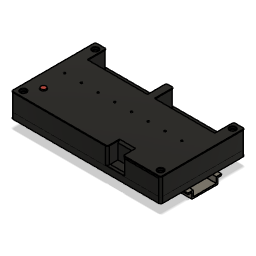
RelayBoardMount (Autodesk Fusion 360 design; units mm, degrees)
Autodesk Fusion 360 part; units mm, degrees
sketch "Skizze1" plane through (0, 0, 0) normal (1, 0, 0) x (0, 0, -1) in component "Rail"
  line L0 (-17.5, 0) -> (17.5, 0)
  line L1 (-13.5, -7.5) -> (13.5, -7.5)
  line L2 (0, -7.5) -> (0, 0) construction
  line L3 (-17.5, 0) -> (-17.5, -1.5)
  line L4 (17.5, 0) -> (17.5, -1.5)
  line L5 (13.5, -7.5) -> (13.5, -1.5)
  line L6 (13.5, -1.5) -> (17.5, -1.5)
  line L7 (-17.5, -1.5) -> (-13.5, -1.5)
  line L8 (-13.5, -1.5) -> (-13.5, -7.5)
  line L9 (-12, 0) -> (-12, -6)
  line L10 (-12, -6) -> (12, -6)
  line L11 (12, -6) -> (12, 0)
  dimension "d1" = 35
  dimension "d2" = 27
  dimension "d3" = 1.5
  dimension "d5" = 7.5
  dimension "d6" = 1.5
  dimension "d7" = 1.5
  dimension "d8" = 1.5
  constraint horizontal L0
  constraint midpoint L2.end L0
  constraint horizontal L1
  constraint midpoint L1 L2.start
  constraint coincident L2.end origin
  constraint vertical L2
  constraint perpendicular L0 L3
  constraint perpendicular L0 L4
  constraint perpendicular L1 L5
  constraint perpendicular L4 L6
  constraint perpendicular L5 L7
  constraint perpendicular L7 L8
  constraint equal L3 L4
  constraint coincident L0 L9.start
  constraint perpendicular L0 L9
  constraint perpendicular L5 L10
  constraint coincident L0 L11.end
  constraint perpendicular L0 L11
  measures "d1" distance of L0.start L0.end
  measures "d2" distance of L1.start L1.end
  measures "d3" distance of L0.end L4.end
  measures "d5" distance of L0 L1
  measures "d6" distance of L1 L10
  measures "d7" distance of L8 L9
  measures "d8" distance of L5 L11
extrude "Extrusion1" add sketch "Skizze1" along normal mid plane 160 contours L0 L1 L3 L4 L5 L6 L7 L8 L9 L10 L11 makes body 1 in component "Rail"
sketch "Skizze1 (2)" plane through (0, 0, 0) normal (0, 1, 0) x (1, 0, 0) in component "DinRailMount"
  line L0 (-80, 17.5) -> (80, 17.5)
  line L1 (-80, 12) -> (80, 12)
  line L2 (-80, -12) -> (80, -12)
  line L3 (80, -17.5) -> (-80, -17.5)
  line L4 (0, 17.5) -> (0, -17.5) construction
  line L5 (-5, 17.5) -> (5, 17.5)
  line L6 (5, 17.5) -> (5, 20.5)
  line L7 (5, 20.5) -> (-5, 20.5)
  line L8 (-5, 20.5) -> (-5, 17.5)
  arc A0 (0, 17.5) -> (0, 11.5) centre (0, 14.5) ccw
  arc A1 (0, 5.5) -> (0, 11.5) centre (0, 8.5) ccw
  arc A2 (0, 5.5) -> (0, -0.5) centre (0, 2.5) ccw
  arc A3 (0, -6.5) -> (0, -0.5) centre (0, -3.5) ccw
  arc A4 (0, -5.8) -> (0, -1.2) centre (0, -3.5) ccw
  arc A5 (0, 6.2) -> (0, -1.2) centre (0, 2.5) ccw
  arc A6 (0, 6.2) -> (0, 10.8) centre (0, 8.5) ccw
  arc A7 (0, 18.2) -> (0, 10.8) centre (0, 14.5) ccw
  arc A8 (0, 16.8) -> (0, 12.2) centre (0, 14.5) ccw
  arc A9 (0, 4.8) -> (0, 12.2) centre (0, 8.5) ccw
  arc A10 (0, 4.8) -> (0, 0.2) centre (0, 2.5) ccw
  arc A11 (0, -7.2) -> (0, 0.2) centre (0, -3.5) ccw
  arc A12 (0, 16.8) -> (5, 17.5) centre (0, 35.0071) ccw
  line L9 (-8.5, 22.5) -> (8.5, 22.5) construction
  line L10 (8.5, 22.5) -> (8.5, -20.5)
  line L11 (8.5, -20.5) -> (-8.5, -20.5)
  line L12 (-8.5, -20.5) -> (-8.5, 22.5)
  line L13 (0, -17.5) -> (0, -20.5) construction
  line L14 (-5.5, 22.5) -> (5.5, 22.5)
  line L15 (5.5, 22.5) -> (5.5, -6.5)
  line L16 (5.5, -6.5) -> (-5.5, -6.5)
  line L17 (-5.5, -6.5) -> (-5.5, 22.5)
  arc A13 (0, -5.8) -> (-5.5, -6.5) centre (0, -27.7571) ccw
  line L18 (8.5, 22.5) -> (8.5, 30.5)
  line L19 (8.5, 30.5) -> (-8.5, 30.5)
  line L20 (-8.5, 30.5) -> (-8.5, 22.5)
  line L21 (0, 30.5) -> (0, 22.5) construction
  circle A14 centre (0, 26.5) radius 1.75
  circle A15 centre (0, -9.5) radius 1.75
  dimension "d89" = 10
  dimension "d91" = 3
  dimension "d94" = 3
  dimension "d95" = 6
  dimension "d98" = 0
  dimension "d99" = -12
  dimension "d100" = 0.7
  dimension "d101" = -0.7
  dimension "d102" = 5
  dimension "d103" = 3
  dimension "d105" = 2
  dimension "d106" = 3.5
  dimension "d107" = 4
  dimension "d108" = 3
  dimension "d111" = 0.5
  dimension "d149" = 3
  constraint midpoint L0 L4.start
  constraint midpoint L3 L4.end
  constraint horizontal L5
  constraint vertical L6
  constraint horizontal L7
  constraint vertical L8
  constraint coincident L0 L5.start
  constraint midpoint L4.start L5
  constraint coincident L4 A0.end
  constraint coincident L4 A0.centre
  constraint coincident L4 A1.start
  constraint coincident L4 A1.centre
  constraint tangent A8 A12
  constraint horizontal L9
  constraint vertical L10
  constraint horizontal L11
  constraint vertical L12
  constraint midpoint L11 L13.end
  constraint collinear L4 L13
  constraint horizontal L14
  constraint vertical L15
  constraint horizontal L16
  constraint vertical L17
  constraint midpoint A3.start L16
  constraint tangent A4 A13
  constraint vertical L18
  constraint horizontal L19
  constraint vertical L20
  constraint coincident L9.end L10.start
  constraint midpoint L19 L21.start
  constraint midpoint L21 A14.centre
  constraint midpoint L14 L21.end
  constraint coincident L4 A15.centre
  constraint equal A14 A15
  measures "d89" distance of L5.start L5.end
  measures "d91" distance of L5.end L6.end
  measures "d94" distance of L5 A0.centre
  measures "d95" distance of A0.centre A1.centre
  measures "d102" distance of L0 L9
  measures "d103" distance of L3 L11
  measures "d105" distance of L7 L14
  measures "d106" diameter of A14
  measures "d107" distance of L19 A14.centre
  measures "d108" distance of L16 A15.centre
  measures "d111" distance of L8 L17
  measures "d149" distance of L12 L17
extrude "Extrusion1'" add sketch "Skizze1 (2)" along normal blind 3 separate body contours L0 L5 L6 L7 L8 | L0 L1 L5 A0 A7 | L0 L1 L5 A0 A8 A9 A12 | L1 A0 A1 A2 A3 A4 A5 A6 A7 L16 A13 | L1 A0 A1 A2 A3 A9 A10 A11 L16 | L0 L10 L12 L14 L15 L17 L18 L19 L20 | L0 L1 L10 L15 | L1 L2 L10 L12 L15 L16 L17 | L0 L1 L12 L17 | L2 L3 L10 L12 | L3 L10 L11 L12 makes body 2 in component "DinRailMount"
sketch "Skizze2" plane through (0, 3, 0) normal (0, 1, 0) x (-1, 0, 0) in component "DinRailMount"
  circle A0 centre (0, -26.5) radius 1.75
  circle A1 centre (0, 9.5) radius 1.75
  line L0 (5.5, 6.5) -> (5.5, -22.5)
  line L1 (5.5, -22.5) -> (-5.5, -22.5)
  line L2 (-5.5, -22.5) -> (-5.5, 6.5)
  line L3 (-5.5, 6.5) -> (-2.1656, 6.5)
  line L4 (-8.5, 20.5) -> (-8.5, -30.5)
  line L5 (-8.5, -30.5) -> (8.5, -30.5)
  line L6 (8.5, -30.5) -> (8.5, 20.5)
  line L7 (8.5, 20.5) -> (-8.5, 20.5)
  line L8 (5, -17.5) -> (6, -17.5)
  line L9 (6, -17.5) -> (6, -22)
  line L10 (6, -22) -> (5.5, -22)
  line L11 (5, -20.5) -> (6, -20.5)
  line L12 (5, -17) -> (6.5, -17)
  line L13 (6.5, -17) -> (6.5, -22.5)
  line L14 (6.5, -22.5) -> (5.5, -22.5)
  line L15 (-5, -17.5) -> (-6, -17.5)
  line L16 (-6, -17.5) -> (-6, -22)
  line L17 (-6, -22) -> (-5.5, -22)
  line L18 (-5, -20.5) -> (-6, -20.5)
  line L19 (-5, -17) -> (-6.5, -17)
  line L20 (-6.5, -17) -> (-6.5, -22.5)
  line L21 (-6.5, -22.5) -> (-5.5, -22.5)
  line L22 (5, -20.5) -> (5, -17.5)
  line L23 (5, -17.5) -> (2.1656, -17.5)
  line L24 (-5, -17.5) -> (-5, -20.5)
  line L25 (-5, -20.5) -> (5, -20.5)
  line L26 (-5, -17.5) -> (-5, -20.5)
  line L27 (-5, -20.5) -> (5, -20.5)
  line L28 (5, -20.5) -> (5, -17.5)
  line L29 (5, -17.5) -> (2.1656, -17.5)
  line L30 (-8.5, 20.5) -> (-8.5, -30.5)
  line L31 (-8.5, -30.5) -> (8.5, -30.5)
  line L32 (8.5, -30.5) -> (8.5, 20.5)
  line L33 (8.5, 20.5) -> (-8.5, 20.5)
  circle A2 centre (0, 9.5) radius 1.75
  circle A3 centre (0, -26.5) radius 1.75
  line L34 (5.5, 6.5) -> (5.5, -22.5)
  line L35 (5.5, -22.5) -> (-5.5, -22.5)
  line L36 (-5.5, -22.5) -> (-5.5, 6.5)
  line L37 (-5.5, 6.5) -> (-2.1656, 6.5)
  arc A4 (0, -4.8) -> (0, -12.2) centre (0, -8.5) ccw
  arc A5 (0, -16.8) -> (0, -12.2) centre (0, -14.5) ccw
  arc A6 (0, -16.8) -> (-5, -17.5) centre (0, -35.0071) ccw
  arc A7 (2.1656, -17.5) -> (0, -10.8) centre (0, -14.5) ccw
  arc A8 (0, -6.2) -> (0, -10.8) centre (0, -8.5) ccw
  arc A9 (0, -6.2) -> (0, 1.2) centre (0, -2.5) ccw
  arc A10 (0, 5.8) -> (0, 1.2) centre (0, 3.5) ccw
  arc A11 (0, 5.8) -> (5.5, 6.5) centre (0, 27.7571) ccw
  arc A12 (-2.1656, 6.5) -> (0, -0.2) centre (0, 3.5) ccw
  arc A13 (0, -4.8) -> (0, -0.2) centre (0, -2.5) ccw
  arc A14 (0, -4.8) -> (0, -12.2) centre (0, -8.5) ccw
  arc A15 (0, -16.8) -> (0, -12.2) centre (0, -14.5) ccw
  arc A16 (0, -16.8) -> (-5, -17.5) centre (0, -35.0071) ccw
  arc A17 (2.1656, -17.5) -> (0, -10.8) centre (0, -14.5) ccw
  arc A18 (0, -6.2) -> (0, -10.8) centre (0, -8.5) ccw
  arc A19 (0, -6.2) -> (0, 1.2) centre (0, -2.5) ccw
  arc A20 (0, 5.8) -> (0, 1.2) centre (0, 3.5) ccw
  arc A21 (0, 5.8) -> (5.5, 6.5) centre (0, 27.7571) ccw
  arc A22 (-2.1656, 6.5) -> (0, -0.2) centre (0, 3.5) ccw
  arc A23 (0, -4.8) -> (0, -0.2) centre (0, -2.5) ccw
  dimension "d119" = 0.5
  dimension "d120" = -0.5
  dimension "d121" = 0.5
  dimension "d148" = 0.5
  constraint perpendicular L1 L9
  constraint perpendicular L0 L10
  constraint coincident L9 L11.end
  constraint perpendicular L9 L11
  constraint coincident L0 L10.end
  constraint coincident L1 L0.end
  constraint perpendicular L2 L15
  constraint perpendicular L15 L16
  constraint coincident L2 L17.end
  constraint perpendicular L2 L17
  constraint coincident L16 L18.end
  constraint perpendicular L16 L18
  constraint equal L8 L15
  constraint equal L9 L16
  measures "d119" distance of L0 L9
  measures "d121" distance of L1 L10
extrude "Extrusion2" cut sketch "Skizze2" against normal blind 1.4 from surface at -0.5 contours L0 L8 L9 L10 L12 L13 L14 L34 | L0 L9 L10 L11 L34 | L0 L8 L9 L11 L34 | L2 L15 L16 L17 L19 L20 L21 L36 | L2 L16 L17 L18 L36 | L2 L15 L16 L18 L36 bodies 2 in component "DinRailMount"
extrude "Extrusion3" add sketch "Skizze2" along normal blind 1 from surface at -1.7 contours L0 L8 L11 L22 L28 L34 | L0 L8 L9 L11 L34 | L2 L15 L18 L24 L26 L36 | L2 L15 L16 L18 L36 bodies 2 in component "DinRailMount"
sketch "Skizze3" plane through (5, 0, 0) normal (1, 0, 0) x (0, 0, -1) in component "DinRailMount"
  line L0 (20.5, 1.3) -> (17.5, 1.3)
  line L1 (17.5, 0) -> (20.5, 0)
  line L2 (20.5, 0) -> (20.5, 1.3)
  line L3 (-17.5, 0) -> (-17.5, -1.5)
  line L4 (-17.5, -1.5) -> (-13.5, -1.5)
  line L5 (-13.5, -1.5) -> (-13.5, -7.5)
  line L6 (-13.5, -7.5) -> (13.5, -7.5)
  line L7 (13.5, -7.5) -> (13.5, -1.5)
  line L8 (13.5, -1.5) -> (17.5, -1.5)
  line L9 (17.5, -1.5) -> (17.5, 0)
  line L10 (17.5, 0) -> (12, 0)
  line L11 (12, 0) -> (12, -6)
  line L12 (12, -6) -> (-12, -6)
  line L13 (-12, -6) -> (-12, 0)
  line L14 (-12, 0) -> (-17.5, 0)
  line L15 (20.5, 0) -> (20.5, -2)
  line L16 (16, -2) -> (16, -1.5)
  line L17 (16, -2) -> (17, -3)
  line L18 (17, -3) -> (19.5, -3)
  line L19 (19.5, -3) -> (20.5, -2)
  line L20 (20.5, -2) -> (16, -2) construction
  line L21 (17.5, 1.3) -> (17.5, 0)
  dimension "d127" = 1.5
  dimension "d129" = 0.5
  dimension "d130" = 1.5
  dimension "d151" = 45
  dimension "d152" = 45
  constraint coincident L1.end L2.start
  constraint perpendicular L1 L15
  constraint coincident L8 L16.end
  constraint perpendicular L8 L16
  constraint horizontal L18
  constraint perpendicular L16 L20
  measures "d127" distance of L9 L16
  measures "d129" distance of L16.start L16.end
  measures "d130" distance of L8 L18
  measures "d151" angle of L17 L20
  measures "d152" angle of L19 L20
extrude "Extrusion4" add sketch "Skizze3" against normal up to surface (10 mm away) contours L1 L8 L9 L15 L16 L17 L18 L19 bodies 2 in component "DinRailMount"
sketch "Skizze4" plane through (8.5, 0, 0) normal (1, 0, 0) x (0, 0, -1) in component "DinRailMount"
  line L0 (-20.5, 0) -> (30.5, 0)
  line L1 (30.5, 0) -> (30.5, 3)
  line L2 (30.5, 3) -> (-20.5, 3)
  line L3 (-20.5, 3) -> (-20.5, 0)
  line L4 (-17.5, 0) -> (-17.5, -1.5)
  line L5 (-17.5, -1.5) -> (-13.5, -1.5)
  line L6 (-13.5, -1.5) -> (-13.5, -7.5)
  line L7 (-13.5, -7.5) -> (13.5, -7.5)
  line L8 (13.5, -7.5) -> (13.5, -1.5)
  line L9 (13.5, -1.5) -> (17.5, -1.5)
  line L10 (17.5, -1.5) -> (17.5, 0)
  line L11 (17.5, 0) -> (12, 0)
  line L12 (12, 0) -> (12, -6)
  line L13 (12, -6) -> (-12, -6)
  line L14 (-12, -6) -> (-12, 0)
  line L15 (-12, 0) -> (-17.5, 0)
  line L16 (-20.5, 0) -> (-20.5, -2)
  line L17 (-19.5, -3) -> (-20.5, -2)
  line L18 (-17, -3) -> (-19.5, -3)
  line L19 (-16, -2) -> (-17, -3)
  line L20 (-16, -2) -> (-16, -1.5)
  line L21 (-16, -2) -> (-20.5, -2) construction
  dimension "d141" = 0.5
  dimension "d143" = 1.5
  dimension "d144" = 1.5
  dimension "d153" = 45
  dimension "d154" = 45
  constraint coincident L0 L3.end
  constraint coincident L0.start L3.end
  constraint coincident L5 L20.end
  constraint perpendicular L5 L20
  constraint perpendicular L0 L16
  constraint perpendicular L20 L21
  measures "d141" distance of L19.start L20.end
  measures "d143" distance of L5 L18
  measures "d144" distance of L4 L20
  measures "d153" angle of L17 L21
  measures "d154" angle of L19 L21
extrude "Extrusion5" add sketch "Skizze4" against normal up to surface (17 mm away) contours L0 L4 L5 L16 L17 L18 L19 L20 bodies 2 in component "DinRailMount"
chamfer "Fase1" distance 1 angle 45 2 edges at (-1.6316, 0, -27.1328) (-1.6316, 0, 8.8672) on bodies 2 in component "DinRailMount"
ref_plane "Arbeitsebene1" through (0, 2, -5) normal (0, 1, 0) x (1, 0, 0) in component "DinRailMount"
sketch "Skizze2 (2)" plane through (0, 2, 0) normal (0, 1, 0) x (1, 0, 0) in component "RelayBottom"
  line L0 (-74, 40) -> (74, 40)
  line L1 (74, 40) -> (74, -40)
  line L2 (74, -40) -> (-74, -40)
  line L3 (-74, -40) -> (-74, 40)
  line L4 (-74, 40) -> (74, -40) construction
  line L5 (74, 40) -> (-74, -40) construction
  line L6 (-77, 43) -> (77, 43)
  line L7 (77, 43) -> (77, -43)
  line L8 (77, -43) -> (-77, -43)
  line L9 (-77, -43) -> (-77, 43)
  circle A0 centre (-71.5, 37.5) radius 2
  line L10 (71.5, -37.5) -> (-71.5, -37.5) construction
  line L11 (-71.5, -37.5) -> (-71.5, 37.5) construction
  line L12 (-71.5, 37.5) -> (71.5, 37.5) construction
  line L13 (71.5, 37.5) -> (71.5, -37.5) construction
  line L14 (71.5, -37.5) -> (-71.5, 37.5) construction
  line L15 (-71.5, -37.5) -> (71.5, 37.5) construction
  circle A1 centre (71.5, 37.5) radius 2
  circle A2 centre (71.5, -37.5) radius 2
  circle A3 centre (-71.5, -37.5) radius 2
  line L16 (-68.5, 39.2321) -> (-71.5, 40.9641)
  line L17 (-71.5, 40.9641) -> (-74.5, 39.2321)
  line L18 (-74.5, 39.2321) -> (-74.5, 35.7679)
  line L19 (-74.5, 35.7679) -> (-71.5, 34.0359)
  line L20 (-71.5, 34.0359) -> (-68.5, 35.7679)
  line L21 (-68.5, 35.7679) -> (-68.5, 39.2321)
  line L22 (-68.5, 39.2321) -> (-68.5, 43)
  line L23 (-74.5, 39.2321) -> (-74.5, 43)
  line L24 (74.5, 35.7679) -> (74.5, 39.2321)
  line L25 (74.5, 39.2321) -> (71.5, 40.9641)
  line L26 (71.5, 40.9641) -> (68.5, 39.2321)
  line L27 (68.5, 39.2321) -> (68.5, 35.7679)
  line L28 (68.5, 35.7679) -> (71.5, 34.0359)
  line L29 (71.5, 34.0359) -> (74.5, 35.7679)
  line L30 (74.5, -35.7679) -> (71.5, -34.0359)
  line L31 (71.5, -34.0359) -> (68.5, -35.7679)
  line L32 (68.5, -35.7679) -> (68.5, -39.2321)
  line L33 (68.5, -39.2321) -> (71.5, -40.9641)
  line L34 (71.5, -40.9641) -> (74.5, -39.2321)
  line L35 (74.5, -39.2321) -> (74.5, -35.7679)
  line L36 (-68.5, -35.7679) -> (-71.5, -34.0359)
  line L37 (-71.5, -34.0359) -> (-74.5, -35.7679)
  line L38 (-74.5, -35.7679) -> (-74.5, -39.2321)
  line L39 (-74.5, -39.2321) -> (-71.5, -40.9641)
  line L40 (-71.5, -40.9641) -> (-68.5, -39.2321)
  line L41 (-68.5, -39.2321) -> (-68.5, -35.7679)
  line L42 (-74.5, -39.2321) -> (-74.5, -43)
  line L43 (-68.5, -39.2321) -> (-68.5, -43)
  line L44 (68.5, -39.2321) -> (68.5, -43)
  line L45 (74.5, -39.2321) -> (74.5, -43)
  line L46 (68.5, 39.2321) -> (68.5, 43)
  line L47 (74.5, 39.2321) -> (74.5, 43)
  line L48 (66.5, -39.2321) -> (66.5, -43)
  line L49 (66.5, -34.6132) -> (66.5, -39.2321)
  line L50 (71.5, -31.7265) -> (66.5, -34.6132)
  line L51 (76.5, -34.6132) -> (71.5, -31.7265)
  line L52 (76.5, -39.2321) -> (76.5, -34.6132)
  line L53 (76.5, -39.2321) -> (76.5, -43)
  line L54 (76.5, 39.2321) -> (76.5, 43)
  line L55 (76.5, 34.6132) -> (76.5, 39.2321)
  line L56 (71.5, 31.7265) -> (76.5, 34.6132)
  line L57 (66.5, 34.6132) -> (71.5, 31.7265)
  line L58 (66.5, 39.2321) -> (66.5, 34.6132)
  line L59 (66.5, 39.2321) -> (66.5, 43)
  line L60 (-66.5, 39.2321) -> (-66.5, 43)
  line L61 (-66.5, 34.6132) -> (-66.5, 39.2321)
  line L62 (-71.5, 31.7265) -> (-66.5, 34.6132)
  line L63 (-76.5, 34.6132) -> (-71.5, 31.7265)
  line L64 (-76.5, 39.2321) -> (-76.5, 34.6132)
  line L65 (-76.5, 39.2321) -> (-76.5, 43)
  line L66 (-76.5, -39.2321) -> (-76.5, -43)
  line L67 (-76.5, -34.6132) -> (-76.5, -39.2321)
  line L68 (-71.5, -31.7265) -> (-76.5, -34.6132)
  line L69 (-66.5, -34.6132) -> (-71.5, -31.7265)
  line L70 (-66.5, -39.2321) -> (-66.5, -34.6132)
  line L71 (-66.5, -39.2321) -> (-66.5, -43)
  point P0 (-71.5, 37.5)
  point P1 (71.5, 37.5)
  point P2 (71.5, -37.5)
  point P3 (-71.5, -37.5)
  dimension "d21" = 148
  dimension "d22" = 80
  dimension "d23" = -3
  dimension "d26" = 4
  dimension "d28" = 2.5
  dimension "d29" = 2.5
  dimension "d31" = 6
  dimension "d35" = 2
  dimension "d36" = 2
  dimension "d37" = -2
  dimension "d38" = 2
  constraint horizontal L0
  constraint perpendicular L0 L1
  constraint parallel L0 L2
  constraint parallel L1 L3
  constraint coincident L4 origin
  constraint coincident L5 origin
  constraint horizontal L10
  constraint perpendicular L10 L11
  constraint parallel L10 L12
  constraint parallel L11 L13
  constraint coincident L14 origin
  constraint coincident L15 origin
  constraint coincident P0 A0.centre
  constraint coincident P1 L12.end
  constraint coincident P2 L10.start
  constraint coincident P3 L10.end
  constraint equal A0 A3
  constraint equal A0 A2
  constraint equal A0 A1
  constraint coincident L6 L22.end
  constraint perpendicular L6 L22
  constraint coincident L6 L23.end
  constraint perpendicular L6 L23
  constraint collinear L21 L22
  constraint equal L21 L26
  constraint equal L21 L32
  constraint equal L21 L41
  constraint coincident L8 L42.end
  constraint parallel L38 L42
  constraint perpendicular L8 L42
  constraint coincident L8 L43.end
  constraint perpendicular L8 L43
  constraint coincident L8 L44.end
  constraint perpendicular L8 L44
  constraint collinear L32 L44
  constraint coincident L8 L45.end
  constraint perpendicular L8 L45
  constraint coincident L6 L46.end
  constraint perpendicular L6 L46
  constraint collinear L27 L46
  constraint coincident L6 L47.end
  constraint perpendicular L6 L47
  measures "d21" distance of L1.end L2.end
  measures "d22" distance of L0.end L1.end
  measures "d26" diameter of A0
  measures "d28" distance of L1 L13
  measures "d29" distance of L2 L10
  measures "d31" distance of L18 L21
extrude "Extrusion2'" add sketch "Skizze2 (2)" along normal blind 2 separate body contours L0 L3 L6 L16 L17 L22 L23 | L0 L3 L17 | L0 L16 L17 | L0 L3 L16 L17 L19 L20 L21 | L3 L17 L18 L19 | L0 L16 L22 | L0 L3 L19 L20 L21 L22 L60 L61 L62 L63 | L3 L6 L18 L19 L23 L63 L64 L65 | L0 L6 L22 L60 | L0 L1 L2 L3 L48 L49 L50 L51 L56 L57 L58 L59 L60 L61 L62 L63 L68 L69 L70 L71 | L3 L6 L8 L9 L63 L64 L65 L66 L67 L68 | L0 L6 L59 L60 | L2 L3 L36 L37 L41 L43 L68 L69 L70 L71 | L3 L8 L37 L38 L42 L66 L67 L68 | L0 L6 L46 L59 | L0 L1 L27 L28 L29 L46 L56 L57 L58 L59 | L2 L3 L36 L37 L39 L40 L41 | L3 L37 L38 L39 | L0 L1 L6 L25 L26 L46 L47 | L0 L26 L46 | L2 L3 L39 | L2 L3 L8 L39 L40 L42 L43 | L0 L25 L26 | L0 L1 L25 L26 L27 L28 L29 | L2 L39 L40 | L0 L1 L25 | L1 L6 L24 L29 L47 L54 L55 L56 | L2 L40 L43 | L2 L8 L43 L71 | L2 L8 L48 L71 | L1 L24 L25 L29 | L1 L6 L7 L8 L51 L52 L53 L54 L55 L56 | L1 L2 L30 L31 L32 L44 L48 L49 L50 L51 | L2 L8 L44 L48 | L1 L8 L30 L35 L45 L51 L52 L53 | L2 L33 L44 | L1 L2 L8 L33 L34 L44 L45 | L1 L30 L34 L35 | L1 L2 L30 L31 L32 L33 L34 | L2 L33 L34 | L1 L2 L34 | A0 | A1 | A2 | A3 makes body 3 in component "RelayBottom"
extrude "Extrusion4'" add sketch "Skizze2 (2)" along normal blind 4 from surface at 2 contours L0 L3 L6 L16 L17 L22 L23 | L0 L3 L17 | L0 L16 L17 | L0 L3 L16 L17 L19 L20 L21 | L3 L17 L18 L19 | L0 L16 L22 | L0 L3 L19 L20 L21 L22 L60 L61 L62 L63 | L3 L6 L18 L19 L23 L63 L64 L65 | L0 L6 L22 L60 | L3 L6 L8 L9 L63 L64 L65 L66 L67 L68 | L0 L6 L59 L60 | L2 L3 L36 L37 L41 L43 L68 L69 L70 L71 | L3 L8 L37 L38 L42 L66 L67 L68 | L0 L6 L46 L59 | L0 L1 L27 L28 L29 L46 L56 L57 L58 L59 | L2 L3 L36 L37 L39 L40 L41 | L3 L37 L38 L39 | L0 L1 L6 L25 L26 L46 L47 | L0 L26 L46 | L2 L3 L39 | L2 L3 L8 L39 L40 L42 L43 | L0 L25 L26 | L0 L1 L25 L26 L27 L28 L29 | L2 L39 L40 | L0 L1 L25 | L1 L6 L24 L29 L47 L54 L55 L56 | L2 L40 L43 | L2 L8 L43 L71 | L2 L8 L48 L71 | L1 L24 L25 L29 | L1 L6 L7 L8 L51 L52 L53 L54 L55 L56 | L1 L2 L30 L31 L32 L44 L48 L49 L50 L51 | L2 L8 L44 L48 | L1 L8 L30 L35 L45 L51 L52 L53 | L2 L33 L44 | L1 L2 L8 L33 L34 L44 L45 | L1 L30 L34 L35 | L1 L2 L30 L31 L32 L33 L34 | L2 L33 L34 | L1 L2 L34 bodies 3 in component "RelayBottom"
extrude "Extrusion3'" cut sketch "Skizze2 (2)" along normal blind 3 from surface at 1.5 contours L0 L3 L6 L16 L17 L22 L23 | L0 L3 L17 | L0 L16 L17 | L0 L3 L16 L17 L19 L20 L21 | L3 L17 L18 L19 | L0 L16 L22 | L2 L3 L36 L37 L39 L40 L41 | L3 L37 L38 L39 | L0 L1 L6 L25 L26 L46 L47 | L0 L26 L46 | L2 L3 L39 | L2 L3 L8 L39 L40 L42 L43 | L0 L25 L26 | L0 L1 L25 L26 L27 L28 L29 | L2 L39 L40 | L0 L1 L25 | L2 L40 L43 | L1 L24 L25 L29 | L2 L33 L44 | L1 L2 L8 L33 L34 L44 L45 | L1 L30 L34 L35 | L1 L2 L30 L31 L32 L33 L34 | L2 L33 L34 | L1 L2 L34 | A0 | A1 | A2 | A3 bodies 3 in component "RelayBottom"
sketch "Skizze4 (2)" plane through (0, 2, 0) normal (0, -1, 0) x (1, 0, 0) in component "RelayBottom"
  line L0 (77, 43) -> (-77, 43)
  line L1 (-77, 43) -> (-77, -43)
  line L2 (-77, -43) -> (77, -43)
  line L3 (77, -43) -> (77, 43)
  line L4 (-77, 0) -> (-47, 0) construction
  line L5 (77, 0) -> (47, 0) construction
  dimension "d158" = 30
  constraint midpoint L1 L4.start
  constraint perpendicular L1 L4
  constraint midpoint L3 L5.start
  constraint perpendicular L3 L5
  constraint equal L4 L5
  measures "d158" distance of L4.start L4.end
sketch "Skizze5" plane through (0, 2, 0) normal (0, -1, 0) x (1, 0, 0) in component "RelayBottom"
  line L0 (77, 43) -> (-77, 43)
  line L1 (-77, 43) -> (-77, -43)
  line L2 (-77, -43) -> (77, -43)
  line L3 (77, -43) -> (77, 43)
  line L4 (-41.5, 6.5) -> (-44.8344, 6.5)
  line L5 (-52.5, 6.5) -> (-52.5, -22.5)
  line L6 (-52.5, -22.5) -> (-41.5, -22.5)
  line L7 (-41.5, -22.5) -> (-41.5, 6.5)
  circle A0 centre (-47, -26.5) radius 1.75
  circle A1 centre (-47, 9.5) radius 1.75
  line L8 (-38.5, 20.5) -> (-38.5, -30.5)
  line L9 (-38.5, -30.5) -> (-55.5, -30.5)
  line L10 (-55.5, -30.5) -> (-55.5, 20.5)
  line L11 (-55.5, 20.5) -> (-38.5, 20.5)
  line L12 (52.5, 7) -> (49.1656, 7)
  line L13 (41.5, 7) -> (41.5, -22)
  line L14 (41.5, -22) -> (52.5, -22)
  line L15 (52.5, -22) -> (52.5, 7)
  circle A2 centre (47, -26) radius 1.75
  circle A3 centre (47, 10) radius 1.75
  line L16 (55.5, 21) -> (55.5, -30)
  line L17 (55.5, -30) -> (38.5, -30)
  line L18 (38.5, -30) -> (38.5, 21)
  line L19 (38.5, 21) -> (55.5, 21)
  line L20 (-38.1, -30.9) -> (-55.9, -30.9)
  line L21 (-55.9, -30.9) -> (-55.9, 20.9)
  line L22 (-55.9, 20.9) -> (-38.1, 20.9)
  line L23 (-38.1, 20.9) -> (-38.1, -30.9)
  line L24 (55.9, -30.4) -> (38.1, -30.4)
  line L25 (38.1, -30.4) -> (38.1, 21.4)
  line L26 (38.1, 21.4) -> (55.9, 21.4)
  line L27 (55.9, 21.4) -> (55.9, -30.4)
  line L28 (-42, -17.5) -> (-42, -20.5)
  line L29 (-42, -20.5) -> (-52, -20.5)
  line L30 (-52, -20.5) -> (-52, -17.5)
  line L31 (-52, -17.5) -> (-49.1656, -17.5)
  line L32 (52, -17) -> (52, -20)
  line L33 (52, -20) -> (42, -20)
  line L34 (42, -20) -> (42, -17)
  line L35 (42, -17) -> (44.8344, -17)
  arc A4 (-47, -10.8) -> (-47, -6.2) centre (-47, -8.5) ccw
  arc A5 (-47, 1.2) -> (-47, -6.2) centre (-47, -2.5) ccw
  arc A6 (-47, 1.2) -> (-47, 5.8) centre (-47, 3.5) ccw
  arc A7 (-52.5, 6.5) -> (-47, 5.8) centre (-47, 27.7571) ccw
  arc A8 (-47, -0.2) -> (-44.8344, 6.5) centre (-47, 3.5) ccw
  arc A9 (-47, -0.2) -> (-47, -4.8) centre (-47, -2.5) ccw
  arc A10 (-47, -12.2) -> (-47, -4.8) centre (-47, -8.5) ccw
  arc A11 (-47, -12.2) -> (-47, -16.8) centre (-47, -14.5) ccw
  arc A12 (-42, -17.5) -> (-47, -16.8) centre (-47, -35.0071) ccw
  arc A13 (-47, -10.8) -> (-49.1656, -17.5) centre (-47, -14.5) ccw
  arc A14 (47, -10.3) -> (47, -5.7) centre (47, -8) ccw
  arc A15 (47, 1.7) -> (47, -5.7) centre (47, -2) ccw
  arc A16 (47, 1.7) -> (47, 6.3) centre (47, 4) ccw
  arc A17 (41.5, 7) -> (47, 6.3) centre (47, 28.2571) ccw
  arc A18 (47, 0.3) -> (49.1656, 7) centre (47, 4) ccw
  arc A19 (47, 0.3) -> (47, -4.3) centre (47, -2) ccw
  arc A20 (47, -11.7) -> (47, -4.3) centre (47, -8) ccw
  arc A21 (47, -11.7) -> (47, -16.3) centre (47, -14) ccw
  arc A22 (52, -17) -> (47, -16.3) centre (47, -34.5071) ccw
  arc A23 (47, -10.3) -> (44.8344, -17) centre (47, -14) ccw
  dimension "d159" = -0.4
  dimension "d160" = -0.4
extrude "Extrusion8" cut sketch "Skizze5" against normal blind 1 contours L4 L5 L6 L7 L28 L29 L30 L31 A4 A5 A6 A7 A8 A9 A10 A11 A12 A13 | A0 | A1 | L8 L9 L10 L11 | L12 L13 L14 L15 L32 L33 L34 L35 A14 A15 A16 A17 A18 A19 A20 A21 A22 A23 | A2 | A3 | L16 L17 L18 L19 | L20 L21 L22 L23 | L24 L25 L26 L27 bodies 3 in component "RelayBottom"
extrude "Extrusion9" cut sketch "Skizze5" against normal up to surface (2 mm away) contours A0 | A1 | A2 | A3 bodies 3 in component "RelayBottom"
fillet "Abrundung2" radius 1 4 edges at (-77, 5, 43) (77, 5, 43) (77, 5, -43) (-77, 5, -43) on bodies 3 in component "RelayBottom"
chamfer "Fase3" distance 0.4 angle 45 16 edges at (0, 2, -43) (76.7071, 2, -42.7071) (77, 2, 0) (76.7071, 2, 42.7071) (0, 2, 43) (-76.7071, 2, 42.7071) (-77, 2, 0) (-76.7071, 2, -42.7071) (0, 8, -43) (-76.7071, 8, -42.7071) (-77, 8, 0) (-76.7071, 8, 42.7071) (0, 8, 43) (76.7071, 8, 42.7071) (77, 8, 0) (76.7071, 8, -42.7071) on bodies 3 in component "RelayBottom"
chamfer "Fase3" distance 0.4 angle 45 8 edges at (-38.1, 2, -5) (-47, 2, 20.9) (-55.9, 2, -5) (-47, 2, -30.9) (55.9, 2, -4.5) (47, 2, 21.4) (38.1, 2, -4.5) (47, 2, -30.4) on bodies 3 in component "RelayBottom"
sketch "Skizze1 (3)" plane through (0, 8, 0) normal (0, 1, 0) x (-1, 0, 0) in component "RelayTop"
  circle A0 centre (71.5, 37.5) radius 2
  circle A1 centre (-71.5, -37.5) radius 2
  circle A2 centre (-71.5, 37.5) radius 2
  line L0 (-66.5, 40) -> (66.5, 40)
  line L1 (66.5, 40) -> (66.5, 34.6132)
  line L2 (66.5, 34.6132) -> (71.5, 31.7265)
  line L3 (71.5, 31.7265) -> (74, 33.1699)
  line L4 (74, 33.1699) -> (74, -33.1699)
  line L5 (74, -33.1699) -> (71.5, -31.7265)
  line L6 (71.5, -31.7265) -> (66.5, -34.6132)
  line L7 (66.5, -34.6132) -> (66.5, -40)
  line L8 (66.5, -40) -> (-66.5, -40)
  line L9 (-66.5, -40) -> (-66.5, -34.6132)
  line L10 (-66.5, -34.6132) -> (-71.5, -31.7265)
  line L11 (-71.5, -31.7265) -> (-74, -33.1699)
  line L12 (-74, -33.1699) -> (-74, 33.1699)
  line L13 (-74, 33.1699) -> (-71.5, 31.7265)
  line L14 (-71.5, 31.7265) -> (-66.5, 34.6132)
  line L15 (-66.5, 34.6132) -> (-66.5, 40)
  circle A3 centre (71.5, -37.5) radius 2
  line L16 (-76, -42.6) -> (76, -42.6)
  arc A4 (76, -42.6) -> (76.6, -42) centre (76, -42) ccw
  line L17 (76.6, -42) -> (76.6, 42)
  arc A5 (76.6, 42) -> (76, 42.6) centre (76, 42) ccw
  line L18 (76, 42.6) -> (-76, 42.6)
  arc A6 (-76, 42.6) -> (-76.6, 42) centre (-76, 42) ccw
  line L19 (-76.6, 42) -> (-76.6, -42)
  arc A7 (-76.6, -42) -> (-76, -42.6) centre (-76, -42) ccw
  line L20 (-74, -33.1699) -> (-74, 33.1699)
  line L21 (-66.5, 40) -> (66.5, 40)
  line L22 (74, 33.1699) -> (74, -33.1699)
  line L23 (66.5, -40) -> (-66.5, -40)
  line L24 (-66.5, 40) -> (-74, 40)
  line L25 (-74, 40) -> (-74, 33.1699)
  line L26 (66.5, 40) -> (74, 40)
  line L27 (74, 40) -> (74, 33.1699)
  line L28 (74, -33.1699) -> (74, -40)
  line L29 (74, -40) -> (66.5, -40)
  line L30 (-74, -33.1699) -> (-74, -40)
  line L31 (-74, -40) -> (-66.5, -40)
  line L32 (76, 43) -> (-76, 43)
  arc A8 (-76, 43) -> (-77, 42) centre (-76, 42) ccw
  line L33 (-77, 42) -> (-77, -42)
  arc A9 (-77, -42) -> (-76, -43) centre (-76, -42) ccw
  line L34 (-76, -43) -> (76, -43)
  arc A10 (76, -43) -> (77, -42) centre (76, -42) ccw
  line L35 (77, -42) -> (77, 42)
  arc A11 (77, 42) -> (76, 43) centre (76, 42) ccw
  line L36 (-78, 42) -> (-78, -42)
  arc A12 (-78, -42) -> (-76, -44) centre (-76, -42) ccw
  line L37 (-76, -44) -> (76, -44)
  arc A13 (76, -44) -> (78, -42) centre (76, -42) ccw
  line L38 (78, -42) -> (78, 42)
  arc A14 (78, 42) -> (76, 44) centre (76, 42) ccw
  line L39 (76, 44) -> (-76, 44)
  arc A15 (-76, 44) -> (-78, 42) centre (-76, 42) ccw
  line L40 (75, 41) -> (75, 33.1699)
  line L41 (75, 33.1699) -> (75, -33.1699)
  line L42 (75, -33.1699) -> (75, -41)
  line L43 (75, -41) -> (66.5, -41)
  line L44 (66.5, -41) -> (-66.5, -41)
  line L45 (-75, -41) -> (-66.5, -41)
  line L46 (-75, -33.1699) -> (-75, -41)
  line L47 (-75, -33.1699) -> (-75, 33.1699)
  line L48 (-75, 41) -> (-75, 33.1699)
  line L49 (-66.5, 41) -> (-75, 41)
  line L50 (-66.5, 41) -> (66.5, 41)
  line L51 (66.5, 41) -> (75, 41)
  circle A16 centre (71.5, 37.5) radius 2
  circle A17 centre (-71.5, 37.5) radius 2
  circle A18 centre (-71.5, -37.5) radius 2
  circle A19 centre (71.5, -37.5) radius 2
  circle A20 centre (-71.5, -37.5) radius 4
  circle A21 centre (-71.5, 37.5) radius 4
  circle A22 centre (71.5, 37.5) radius 4
  circle A23 centre (71.5, -37.5) radius 4
  line L52 (-77.3, 42) -> (-77.3, -42)
  arc A24 (-77.3, -42) -> (-76, -43.3) centre (-76, -42) ccw
  line L53 (-76, -43.3) -> (76, -43.3)
  arc A25 (76, -43.3) -> (77.3, -42) centre (76, -42) ccw
  line L54 (77.3, -42) -> (77.3, 42)
  arc A26 (77.3, 42) -> (76, 43.3) centre (76, 42) ccw
  line L55 (76, 43.3) -> (-76, 43.3)
  arc A27 (-76, 43.3) -> (-77.3, 42) centre (-76, 42) ccw
  dimension "d167" = 1
  dimension "d168" = -1
  dimension "d169" = 2
  dimension "d170" = 2
  dimension "d171" = 2
  dimension "d172" = 2
  dimension "d178" = 0.3
  constraint coincident L0.start L15.end
  constraint perpendicular L15 L24
  constraint coincident L12.end L13.start
  constraint perpendicular L24 L25
  constraint coincident L0.end L1.start
  constraint perpendicular L1 L26
  constraint coincident L3.end L4.start
  constraint perpendicular L26 L27
  constraint coincident L4.end L5.start
  constraint vertical L28
  constraint coincident L7.end L8.start
  constraint perpendicular L28 L29
  constraint coincident L11.end L12.start
  constraint parallel L12 L30
  constraint coincident L8.end L9.start
  constraint perpendicular L30 L31
  measures "d169" distance of A1
  measures "d170" distance of A2
  measures "d171" distance of A0
  measures "d172" distance of A3
extrude "Extrusion1''" add sketch "Skizze1 (3)" along normal blind 1 separate body contours L49 A21 | L51 A22 | L40 A22 | L48 A21 | L46 A20 | L42 A23 | L43 A23 | L45 A20 | L16 A4 L17 A5 L18 A6 L19 A7 | L32 A8 L33 A9 L34 A10 L35 A11 | L36 A12 L37 A13 L38 A14 L39 A15 | L52 A24 L53 A25 L54 A26 L55 A27 makes body 4 in component "RelayTop"
extrude "Extrusion3''" add sketch "Skizze1 (3)" against normal up to surface (6 mm away) contours L36 A12 L37 A13 L38 A14 L39 A15 bodies 4 in component "RelayTop"
sketch "Skizze3 (2)" plane through (0, 9, 0) normal (0, 1, 0) x (-1, 0, 0) in component "RelayTop"
  line L0 (-75, 41) -> (75, 41)
  line L1 (75, 41) -> (75, 33.1699)
  line L2 (75, 33.1699) -> (75, -41)
  line L3 (75, -41) -> (66.5, -41)
  line L4 (66.5, -41) -> (-66.5, -41)
  line L5 (-66.5, -41) -> (-75, -41)
  line L6 (-75, -41) -> (-75, 41)
  arc A0 (-76, 44) -> (-78, 42) centre (-76, 42) ccw
  line L7 (-78, 42) -> (-78, -42)
  arc A1 (-78, -42) -> (-76, -44) centre (-76, -42) ccw
  line L8 (-76, -44) -> (76, -44)
  arc A2 (76, -44) -> (78, -42) centre (76, -42) ccw
  line L9 (78, -42) -> (78, 42)
  arc A3 (78, 42) -> (76, 44) centre (76, 42) ccw
  line L10 (76, 44) -> (-76, 44)
  circle A4 centre (-71.5, -37.5) radius 2
  line L11 (66.5, -40) -> (-66.5, -40)
  line L12 (-74, -33.1699) -> (-74, 33.1699)
  circle A5 centre (-71.5, 37.5) radius 2
  line L13 (-66.5, 40) -> (66.5, 40)
  circle A6 centre (71.5, 37.5) radius 2
  line L14 (74, 33.1699) -> (74, -33.1699)
  circle A7 centre (71.5, -37.5) radius 2
  circle A8 centre (-71.5, 37.5) radius 4
  circle A9 centre (71.5, 37.5) radius 4
  circle A10 centre (71.5, -37.5) radius 4
  circle A11 centre (-71.5, -37.5) radius 4
  line L15 (-4, -44) -> (4, -44)
  line L16 (0, -44) -> (0, -41) construction
  line L17 (4, -44) -> (4, -26)
  line L18 (4, -26) -> (66, -26)
  line L19 (66, -26) -> (66, -44)
  line L20 (-4, -44) -> (-4, -26)
  line L21 (-4, -26) -> (-66, -26)
  line L22 (-66, -26) -> (-66, -44)
  line L23 (-68, -24) -> (-68, -44)
  line L24 (-2, -24) -> (-68, -24)
  line L25 (-2, -42) -> (-2, -24)
  line L26 (-2, -42) -> (2, -42)
  line L27 (2, -42) -> (2, -24)
  line L28 (2, -24) -> (68, -24)
  line L29 (68, -24) -> (68, -44)
  line L30 (-38.5, 44) -> (-38.5, 33)
  line L31 (-38.5, 33) -> (-22.5, 33)
  line L32 (-22.5, 33) -> (-22.5, 44)
  line L33 (-40.5, 44) -> (-40.5, 31)
  line L34 (-40.5, 31) -> (-20.5, 31)
  line L35 (-20.5, 31) -> (-20.5, 44)
  dimension "d189" = 2
  dimension "d190" = 2
  dimension "d191" = 2
  dimension "d192" = 2
  dimension "d193" = 14
  dimension "d194" = 8
  dimension "d195" = 8
  dimension "d196" = 2
  dimension "d203" = 16
  dimension "d204" = 35.5
  dimension "d205" = 11
  dimension "d206" = 2
  constraint coincident L8 L15.start
  constraint coincident L8 L15.end
  constraint midpoint L15 L16.start
  constraint midpoint L4 L16.end
  constraint perpendicular L15 L16
  constraint perpendicular L15 L17
  constraint perpendicular L17 L18
  constraint coincident L8 L19.end
  constraint perpendicular L8 L19
  constraint perpendicular L15 L20
  constraint perpendicular L20 L21
  constraint coincident L8 L22.end
  constraint perpendicular L8 L22
  constraint collinear L18 L21
  constraint equal L18 L21
  constraint coincident L10 L30.start
  constraint perpendicular L0 L30
  constraint perpendicular L30 L31
  constraint coincident L10 L32.end
  constraint perpendicular L10 L32
  measures "d189" distance of A5
  measures "d190" distance of A6
  measures "d191" distance of A7
  measures "d192" distance of A4
  measures "d193" distance of L11 L21
  measures "d194" distance of L12 L22
  measures "d195" distance of L15.start L15.end
  measures "d203" distance of L30.end L31.end
  measures "d204" distance of L12 L30
  measures "d205" distance of L31.end L32.end
extrude "Extrusion4''" add sketch "Skizze3 (2)" along normal blind 15.5 contours L0 L5 L6 A0 L7 A1 L8 L10 A8 A11 L23 L33 | L0 L6 A8 | L0 A8 | L0 L6 A8 | L6 A8 | L0 L10 L30 L33 | L0 L13 L30 L33 | L5 L6 A11 L23 | L6 A11 | L13 L30 L31 L32 L33 L34 L35 | L5 L6 A11 | L4 L5 L11 A11 L20 L21 L22 L23 L24 L25 | A11 L23 | L0 L10 L32 L35 | L0 L13 L32 L35 | L5 A11 | L5 A11 L23 | L0 L1 L2 L3 L8 A2 L9 A3 L10 A9 A10 L29 L35 | L4 L5 L8 L22 L23 | L0 A9 | L0 L1 A9 | L4 L11 L20 L25 | L4 L11 L25 L27 | L0 L1 A9 | L1 A9 | L3 L4 L11 A10 L17 L18 L19 L27 L28 L29 | L4 L11 L17 L27 | L4 L8 L15 L17 L20 L25 L26 L27 | L4 L25 L26 L27 | L2 A10 | L2 L3 A10 L29 | L2 L3 A10 | A10 L29 | L3 L4 L8 L19 L29 | L3 A10 | L3 A10 L29 bodies 4 in component "RelayTop"
sketch "Skizze4 (3)" plane through (0, 24.5, 0) normal (0, 1, 0) x (-1, 0, 0) in component "RelayTop"
  circle A0 centre (-71.5, -37.5) radius 2
  line L0 (2, -24) -> (2, -40)
  line L1 (2, -40) -> (-2, -40)
  line L2 (-2, -40) -> (-2, -24)
  line L3 (-2, -24) -> (-68, -24)
  line L4 (-68, -24) -> (-68, -35.5635)
  arc A1 (-68, -35.5635) -> (-75, -35.5635) centre (-71.5, -37.5) ccw
  line L5 (-75, -35.5635) -> (-75, 35.5635)
  arc A2 (-75, 35.5635) -> (-69.5635, 41) centre (-71.5, 37.5) ccw
  line L6 (-69.5635, 41) -> (-40.5, 41)
  arc A3 (69.5635, 41) -> (75, 35.5635) centre (71.5, 37.5) ccw
  line L7 (75, 35.5635) -> (75, 33.1699)
  line L8 (75, 33.1699) -> (75, -35.5635)
  arc A4 (75, -35.5635) -> (68, -35.5635) centre (71.5, -37.5) ccw
  line L9 (68, -35.5635) -> (68, -24)
  line L10 (68, -24) -> (2, -24)
  circle A5 centre (71.5, 37.5) radius 2
  circle A6 centre (-71.5, 37.5) radius 2
  circle A7 centre (71.5, -37.5) radius 2
  line L11 (-4, -44) -> (4, -44)
  line L12 (4, -44) -> (4, -26)
  line L13 (4, -26) -> (66, -26)
  line L14 (66, -26) -> (66, -44)
  line L15 (66, -44) -> (76, -44)
  arc A8 (76, -44) -> (78, -42) centre (76, -42) ccw
  line L16 (78, -42) -> (78, 42)
  arc A9 (78, 42) -> (76, 44) centre (76, 42) ccw
  line L17 (-38.5, 44) -> (-76, 44)
  arc A10 (-76, 44) -> (-78, 42) centre (-76, 42) ccw
  line L18 (-78, 42) -> (-78, -42)
  arc A11 (-78, -42) -> (-76, -44) centre (-76, -42) ccw
  line L19 (-76, -44) -> (-66, -44)
  line L20 (-66, -44) -> (-66, -26)
  line L21 (-66, -26) -> (-4, -26)
  line L22 (-4, -26) -> (-4, -44)
  line L23 (-40.5, 41) -> (-40.5, 31)
  line L24 (-40.5, 31) -> (-20.5, 31)
  line L25 (-20.5, 31) -> (-20.5, 41)
  line L26 (-20.5, 41) -> (69.5635, 41)
  line L27 (76, 44) -> (-22.5, 44)
  line L28 (-22.5, 44) -> (-22.5, 33)
  line L29 (-22.5, 33) -> (-38.5, 33)
  line L30 (-38.5, 33) -> (-38.5, 44)
  circle A12 centre (-56, 0) radius 1
  circle A13 centre (-56, 0) radius 3
  line L31 (-74, -33.1699) -> (-74, 33.1699)
  line L32 (66.5, -40) -> (-66.5, -40)
  circle A14 centre (-38.5714, 0) radius 3
  circle A15 centre (-38.5714, 0) radius 1
  circle A16 centre (-21.1429, 0) radius 3
  circle A17 centre (-21.1429, 0) radius 1
  circle A18 centre (-3.7143, 0) radius 3
  circle A19 centre (-3.7143, 0) radius 1
  circle A20 centre (13.7143, 0) radius 3
  circle A21 centre (13.7143, 0) radius 1
  circle A22 centre (31.1429, 0) radius 3
  circle A23 centre (31.1429, 0) radius 1
  circle A24 centre (48.5714, 0) radius 3
  circle A25 centre (48.5714, 0) radius 1
  circle A26 centre (66, 0) radius 3
  circle A27 centre (66, 0) radius 1
  circle A28 centre (63, 25) radius 3
  line L33 (74, 33.1699) -> (74, -33.1699)
  circle A29 centre (63, 25) radius 5
  circle A30 centre (-71.5, -37.5) radius 2.9435
  circle A31 centre (-71.5, 37.5) radius 2.9435
  circle A32 centre (71.5, 37.5) radius 2.9435
  circle A33 centre (71.5, -37.5) radius 2.9435
  dimension "d209" = 2
  dimension "d210" = 2
  dimension "d211" = 18
  dimension "d212" = 40
  dimension "d215" = 122
  dimension "d216" = 0
  dimension "d223" = 6
  dimension "d224" = 11
  dimension "d225" = 16
  dimension "d226" = 2
  dimension "d228" = 5.887
  constraint concentric A12 A13
  constraint concentric A28 A29
  constraint concentric A0 A30
  constraint concentric A2 A31
  constraint concentric A3 A32
  constraint concentric A4 A33
  constraint equal A31 A32
  constraint equal A32 A33
  constraint equal A30 A33
  measures "d209" diameter of A12
  measures "d210" distance of A12 A13
  measures "d211" distance of A12.centre L31
  measures "d212" distance of A12.centre L32
  measures "d223" diameter of A28
  measures "d224" distance of A28.centre L33
  measures "d225" distance of L26 A28.centre
  measures "d226" distance of A28 A29
  measures "d228" diameter of A30
extrude "Extrusion5'" add sketch "Skizze4 (3)" along normal blind 2 contours L0 L2 L3 L4 A1 L5 A2 L6 A3 L7 L8 A4 L9 L10 L12 L13 L14 L15 A8 L16 A9 L17 A10 L18 A11 L19 L20 L21 L22 L23 L24 L25 L26 L27 L28 L29 L30 L32 | L0 L1 L2 L3 L4 A1 L5 A2 L6 A3 L7 L8 A4 L9 L10 L23 L24 L25 L26 L32 | L1 L11 L12 L22 L32 | A13 | A14 | A16 | A18 | A20 | A22 | A24 | A26 | A29 bodies 4 in component "RelayTop"
extrude "Extrusion6" add sketch "Skizze4 (3)" against normal up to surface (14.5 mm away) contours A13 | A14 | A16 | A18 | A20 | A22 | A24 | A26 bodies 4 in component "RelayTop"
extrude "Extrusion7" add sketch "Skizze4 (3)" against normal up to surface (9.5 mm away) contours A29 bodies 4 in component "RelayTop"
chamfer "Fase1'" distance 2 distance2 5 9 edges at (58.797, 24.5, -1.0848) (41.3684, 24.5, -1.0848) (23.9398, 24.5, -1.0848) (6.5113, 24.5, -1.0848) (-10.9173, 24.5, -1.0848) (-28.3459, 24.5, -1.0848) (-45.7744, 24.5, -1.0848) (-63.203, 24.5, -1.0848) (-58.3384, 24.5, 23.1919) measured on face at (-17.459, 24.5, 23.6981) measured on face at (-17.459, 24.5, 23.6981) measured on face at (-17.459, 24.5, 23.6981) measured on face at (-17.459, 24.5, 23.6981) measured on face at (-17.459, 24.5, 23.6981) measured on face at (-17.459, 24.5, 23.6981) measured on face at (-17.459, 24.5, 23.6981) measured on face at (-17.459, 24.5, 23.6981) measured on face at (-17.459, 24.5, 23.6981) on bodies 4 in component "RelayTop"
fillet "Abrundung1" radius 2 4 edges at (66, 17.75, -44) (4, 17.75, -44) (-4, 17.75, -44) (-66, 17.75, -44) on bodies 4 in component "RelayTop"
fillet "Abrundung1" radius 2 3 edges at (38.5, 16.75, 44) (38.5, 25.5, 44) (22.5, 17.75, 44) on bodies 4 in component "RelayTop"
chamfer "Fase2" distance 2 angle 45 3 edges at (35, 26.5, -26) (-35, 26.5, -26) (30.5, 26.5, 33) on bodies 4 in component "RelayTop"
chamfer "Fase3'" distance 0.4 angle 45 23 edges at (66, 26.5, -33) (66.5858, 26.5, -43.4142) (72, 26.5, -44) (77.4142, 26.5, -43.4142) (78, 26.5, 0) (77.4142, 26.5, 43.4142) (58.25, 26.5, 44) (39.0858, 26.5, 43.4142) (38.5, 26.5, 36.5) (22.5, 26.5, 36.5) (21.9142, 26.5, 43.4142) (-27.75, 26.5, 44) (-77.4142, 26.5, 43.4142) (-78, 26.5, 0) (-77.4142, 26.5, -43.4142) (-72, 26.5, -44) (-66.5858, 26.5, -43.4142) (-66, 26.5, -33) (-4, 26.5, -33) (-3.4142, 26.5, -43.4142) (0, 26.5, -44) (3.4142, 26.5, -43.4142) (4, 26.5, -33) on bodies 4 in component "RelayTop"
chamfer "Fase3'" distance 0.4 angle 45 4 edges at (74.2443, 26.5, 38.5644) (74.2443, 26.5, -36.4356) (-68.7557, 26.5, 38.5644) (-68.7557, 26.5, -36.4356) on bodies 4 in component "RelayTop"
sketch "Skizze1 (4)" plane through (0, 15, 0) normal (0, -1, 0) x (1, 0, 0) in component "ResetButton"
  circle A0 centre (-63, 25) radius 3
  circle A1 centre (-63, 25) radius 5
  circle A2 centre (-63, 25) radius 5
  circle A3 centre (-63, 25) radius 3
  circle A4 centre (-63, 25) radius 2.6
  dimension "d233" = -0.4
extrude "Extrusion1'''" add sketch "Skizze1 (4)" along normal blind 1 separate body contours A0 A3 | A1 A2 | A4 makes body 5 in component "ResetButton"
extrude "Extrusion2''" add sketch "Skizze1 (4)" against normal up to surface (12.5 mm away) contours A4 bodies 5 in component "ResetButton"
component "Rail" placed x (1, 0, 0) y (0, 1, 0) z (0, 0, 1) at (0, 0, 0)
component "DinRailMount" placed x (1, 0, 0) y (0, 1, 0) z (0, 0, 1) at (-47, 0, 0)
component "DinRailMount" placed x (1, 0, 0) y (0, 1, 0) z (0, 0, 1) at (47, 0, 0.5)
component "RelayBottom" placed x (1, 0, 0) y (0, 1, 0) z (0, 0, 1) at (0, 0, 0)
component "RelayTop" placed x (1, 0, 0) y (0, 1, 0) z (0, 0, 1) at (0, 0, 0)
component "ResetButton" placed x (1, 0, 0) y (0, 1, 0) z (0, 0, 1) at (0, 0, 0)
